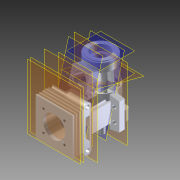
# Autodesk Inventor part: Engine Block
Saved by Autodesk Inventor 2015 (Build 190159000, 159)
## iProperties
Created: 2016-02-24
Part Number: Engine Block
Material: Aluminum 6061-AHC
Document SubType Name: Modeling
Designer: Owner
Density: 2.7 g/cm^3
Appearance: Aluminum - Dark
Author: Owner
Autodesk Inventor part; units mm, degrees
(part 1 of 2)
ref_plane "YZ Plane" through (0, 0, 0) normal (1, 0, 0) x (0, 1, 0)
ref_plane "XZ Plane" through (0, 0, 0) normal (0, 1, 0) x (-1, 0, 0)
sketch "Sketch1" plane through (0, 0, 0) normal (0, 1, 0) x (-1, 0, 0)
  circle A0 centre (0, 0) radius 12.5095
  dimension "d0" = 25.019
  constraints: 1 centre point, 1 coincident
  measures "d0" diameter of A0
extrude "Extrusion1" add sketch "Sketch1" along normal blind 26.162
ref_plane "Work Plane1" through (0, 47.625, 0) normal (0, -1, 0) x (1, 0, 0)
sketch "Sketch2" plane through (0, 47.625, 0) normal (0, -1, 0) x (1, 0, 0)
  circle A0 centre (0, 0) radius 11.049
  dimension "d4" = 22.098
  constraints: 1 centre point, 1 coincident
  measures "d4" diameter of A0
extrude "Extrusion2" add sketch "Sketch2" along normal blind 7.62
sketch "Sketch4" plane through (0, 40.005, 0) normal (0, -1, 0) x (1, 0, 0)
  circle A0 centre (0, 0) radius 7.239
  dimension "d7" = 14.478
  constraints: 1 centre point, 1 coincident
  measures "d7" diameter of A0
sketch "Sketch5" plane through (0, 26.162, 0) normal (0, 1, 0) x (1, 0, 0)
  circle A0 centre (0, 0) radius 8.7122
  dimension "d8" = 17.4244
  constraints: 1 centre point, 1 coincident
  measures "d8" diameter of A0
loft "Loft1" add profiles "Sketch5", "Sketch4"
sketch "Sketch6" plane through (0, 40.005, 0) normal (0, -1, 0) x (1, 0, 0)
  circle A0 centre (0, 0) radius 10.414
  dimension "d13" = 20.828
  constraints: 1 centre point, 1 coincident
  measures "d13" diameter of A0
sketch "Sketch7" plane through (0, 26.162, 0) normal (0, 1, 0) x (1, 0, 0)
  circle A0 centre (0, 0) radius 11.8872
  dimension "d14" = 23.7744
  constraints: 1 centre point, 1 coincident
  measures "d14" diameter of A0
surface_loft "LoftSrf1"
sketch "Sketch8" plane through (0, 0, 0) normal (1, 0, 0) x (0, 1, 0)
  line L0 (47.625, -11.049) -> (40.005, -11.049) construction
  line L1 (40.005, -11.049) -> (40.005, -10.16) construction
  line L2 (40.005, 11.049) -> (40.005, -11.049) construction
  line L3 (40.005, -10.16) -> (26.162, -10.16)
  line L4 (26.162, -12.5095) -> (26.162, 12.5095) projected
  line L5 (40.005, -10.16) -> (40.005, -8.255)
  line L6 (40.005, -8.255) -> (26.162, -8.255)
  line L7 (40.005, -8.255) -> (40.005, -5.08) construction
  line L8 (40.005, -5.08) -> (26.162, -5.08)
  line L9 (26.162, -8.255) -> (26.162, -10.16)
  line L10 (40.005, -5.08) -> (40.005, -3.175)
  line L11 (40.005, -3.175) -> (26.162, -3.175)
  line L12 (26.162, -3.175) -> (26.162, -5.08)
  line L13 (40.005, 0) -> (40.005, 1.905)
  line L14 (40.005, 0) -> (26.162, 0)
  line L15 (26.162, 0) -> (26.162, 1.905)
  line L16 (40.005, 1.905) -> (26.162, 1.905)
  line L17 (40.005, 1.905) -> (40.005, 5.08) construction
  line L18 (40.005, 5.08) -> (26.162, 5.08)
  line L19 (26.162, 5.08) -> (26.162, 6.985)
  line L20 (26.162, 6.985) -> (40.005, 6.985)
  line L21 (40.005, 5.08) -> (40.005, 6.985)
  point P0 (0, 0)
  dimension "d19" = 0.889
  dimension "d20" = 1.905
  dimension "d21" = 3.175
  dimension "d22" = 1.905
  dimension "d23" = 1.905
  dimension "d24" = 3.175
  dimension "d25" = 1.905
  constraints: 38 end point, 6 horizontal, 3 vertical, 1 perpendicular, 1 point on line, 18 other
  measures "d19" distance of L1.start L1.end
  measures "d20" distance of L1.end L5.end
  measures "d21" distance of L5.end L7.end
  measures "d22" distance of L7.end L10.end
  measures "d23" distance of L13.start L13.end
  measures "d24" distance of L13.end L17.end
  measures "d25" distance of L18.end L19.end
extrude "Extrusion3" add sketch "Sketch8" along normal up to surface round surface about axis through (0, 26.162, 0) along (0, 1, 0) radius 11.8872 half angle -6.074668 far side no
mirror "Mirror1" about plane through (0, 0, 0) normal (1, 0, 0) of "Extrusion3"
sketch "Sketch11" plane through (6.1709, 26.162, -10.16) normal (0, 0, -1) x (-1, 0, 0)
  line L0 (12.5196, 13.843) -> (-0.1778, 13.843) projected
  line L1 (6.1709, 13.843) -> (6.1709, 0)
  line L2 (0.964, 0) -> (11.3778, 0) projected
  line L3 (7.4409, 13.843) -> (7.4409, 0)
  line L4 (4.9009, 13.843) -> (4.9009, 0)
  line L5 (4.9009, 13.843) -> (6.1709, 13.843)
  line L6 (6.1709, 13.843) -> (7.4409, 13.843)
  line L7 (6.1709, 0) -> (7.4409, 0)
  line L8 (4.9009, 0) -> (6.1709, 0)
  point P0 (6.1709, -26.162)
  dimension "d30" = 1.27
  dimension "d31" = 1.27
  constraints: 14 end point, 4 collinear, 4 point on line, 2 midpoint, 2 parallel
  measures "d30" distance between parallel lines of L3 L1
  measures "d31" distance between parallel lines of L1 L4
extrude "Extrusion5" add sketch "Sketch11" along normal up to surface from surface at -17.145 round surface about axis through (0, 26.162, 0) along (0, 1, 0) radius 11.8872 half angle -6.074668 far side no
ref_plane "Work Plane2" through (0, 31.75, 0) normal (0, -1, 0) x (1, 0, 0)
ref_plane "Work Plane3" through (0, 31.75, 0) normal (0, -0.258819, -0.9659258) x (1, 0, 0)
ref_plane "Work Plane4" through (0, 31.75, 0) normal (0, 0.9659258, -0.258819) x (1, 0, 0)
ref_plane "Work Plane5" through (0, 0, 20.32) normal (0, 0, 1) x (1, 0, 0)
ref_plane "Work Plane6" through (0, 36.457, 17.5667) normal (0, -0.258819, -0.9659258) x (1, 0, 0)
sketch "Sketch12" plane through (0, 36.457, 17.5667) normal (0, -0.258819, -0.9659258) x (1, 0, 0)
  point P0 (0, 30.6681)
sketch "Sketch13" plane through (0, 36.457, 17.5667) normal (0, -0.258819, -0.9659258) x (1, 0, 0)
  line L0 (-6.985, -6.985) -> (6.985, -6.985)
  line L1 (6.985, -6.985) -> (6.985, 6.985)
  line L2 (6.985, 6.985) -> (-6.985, 6.985)
  line L3 (-6.985, 6.985) -> (-6.985, -6.985)
  line L4 (-6.985, -6.985) -> (6.985, 6.985) construction
  line L5 (6.985, -6.985) -> (-6.985, 6.985) construction
  point P0 (0, 30.6681)
  point P1 (0, 0)
  dimension "d41" = 13.97
  dimension "d42" = 13.97
  constraints: 12 end point, 2 midpoint, 2 parallel, 1 horizontal, 1 perpendicular
  measures "d41" distance of L2.end L1.end
  measures "d42" distance of L1.end L0.end
extrude "Extrusion6" add sketch "Sketch13" along normal up to next
sketch "Sketch14" plane through (0, 0, 0) normal (0, -1, 0) x (1, 0, 0)
  line L0 (9.0932, -9.0932) -> (-9.0932, -9.0932)
  line L1 (-9.0932, -9.0932) -> (-9.0932, 9.0932)
  line L2 (-9.0932, 9.0932) -> (9.0932, 9.0932)
  line L3 (9.0932, 9.0932) -> (9.0932, -9.0932)
  line L4 (9.0932, -9.0932) -> (-9.0932, 9.0932) construction
  line L5 (-9.0932, -9.0932) -> (9.0932, 9.0932) construction
  circle A0 centre (9.0932, -9.0932) radius 3.175
  circle A1 centre (-9.0932, -9.0932) radius 3.175
  circle A2 centre (-9.0932, 9.0932) radius 3.175
  circle A3 centre (9.0932, 9.0932) radius 3.175
  point P0 (0, 0)
  dimension "d45" = 18.1864
  dimension "d46" = 18.1864
  dimension "d47" = 6.35
  dimension "d48" = 6.35
  dimension "d49" = 6.35
  dimension "d50" = 6.35
  constraints: 12 end point, 4 centre point, 4 coincident, 2 midpoint, 2 parallel, 1 horizontal, 1 perpendicular
  measures "d45" distance of L1.end L2.end
  measures "d46" distance of L0.end L1.end
  measures "d47" diameter of A0
  measures "d48" diameter of A1
  measures "d49" diameter of A2
  measures "d50" diameter of A3
extrude "Extrusion7" add sketch "Sketch14" against normal blind 8.128 contours A1 L1 L0 | L0 L1 A1 | A0 L3 L0 | L0 L3 A0 | A2 L2 L1 | L1 L2 A2 | A3 L2 L3 | L3 L2 A3
sketch "Sketch15" plane through (0, 0, 0) normal (0, -1, 0) x (1, 0, 0)
  arc A0 (6.3881, -10.7555) -> (10.7555, -6.3881) centre (9.0932, -9.0932) ccw projected
  arc A1 (-10.7555, -6.3881) -> (-6.3881, -10.7555) centre (-9.0932, -9.0932) ccw projected
  arc A2 (-6.3881, 10.7555) -> (-10.7555, 6.3881) centre (-9.0932, 9.0932) ccw projected
  arc A3 (10.7555, 6.3881) -> (6.3881, 10.7555) centre (9.0932, 9.0932) ccw projected
  point P0 (0, 0)
hole "Hole1" at (9.0932, 0, -9.0932) at (-9.0932, 0, -9.0932) at (-9.0932, 0, 9.0932) at (9.0932, 0, 9.0932) direction (0, 1, 0) diameter 1.9304 depth 5.715 tip angle 118
fillet "Fillet1" radius 5.08 4 edges at (6.3881, 4.064, 10.7555) (-6.3881, 4.064, 10.7555) (-6.3881, 4.064, -10.7555) (6.3881, 4.064, -10.7555)
sketch "Sketch16" plane through (0, 0, 0) normal (0, 0, 1) x (1, 0, 0)
  line L0 (4.0733, 0) -> (4.0733, 8.128) projected
  line L1 (-4.0733, 0) -> (4.0733, 0) projected
  line L2 (-4.0733, 8.128) -> (-4.0733, 0) projected
  line L3 (-4.0733, 8.128) -> (-10.7555, 8.128) projected
  line L4 (-10.7555, 8.128) -> (-10.7555, 0) projected
  line L5 (-10.7555, 0) -> (-10.7555, 0) projected
  line L6 (-10.7555, 0) -> (-10.7555, 8.128) projected
  line L7 (-10.7555, 8.128) -> (-4.0733, 8.128) projected
  line L8 (-4.0733, 0) -> (-4.0733, 8.128) projected
  line L9 (4.0733, 0) -> (-4.0733, 0) projected
  line L10 (4.0733, 8.128) -> (4.0733, 0) projected
  line L11 (4.0733, 8.128) -> (10.7555, 8.128) projected
  line L12 (10.7555, 8.128) -> (10.7555, 0) projected
  line L13 (10.7555, 0) -> (10.7555, 0) projected
  line L14 (10.7555, 0) -> (10.7555, 8.128) projected
  line L15 (10.7555, 8.128) -> (4.0733, 8.128) projected
  line L16 (12.5095, 26.162) -> (-12.5095, 26.162) projected
  line L17 (-12.5095, 0) -> (-12.5095, 26.162) projected
  line L18 (-7.7987, 0) -> (-12.2682, 0) projected
  line L19 (-7.7987, 0) -> (-4.0733, 0) projected
  line L20 (12.5095, 0) -> (12.5095, 26.162) projected
  line L21 (-12.5095, 0) -> (-6.9215, 0)
  line L22 (-6.9215, 0) -> (-6.9215, 26.162)
  line L23 (-7.0779, 26.162) -> (-2.7852, 26.162) projected
  line L24 (-6.9215, 0) -> (-19.4918, 2.2844)
  line L25 (-6.9215, 0) -> (5.8547, 0) construction
  line L26 (-19.4918, 2.2844) -> (-19.4918, 23.8744)
  line L27 (-19.4918, 23.8744) -> (-6.9215, 26.162)
  point P0 (0, 0)
  dimension "d61" = 5.588
  dimension "d62" = 12.7762
  dimension "d63" = 169.7
  dimension "d64" = 21.59
  constraints: 12 end point, 2 point on line, 1 equal length, 1 horizontal, 1 perpendicular, 1 vertical
  measures "d61" distance of L17.start L21.end
  measures "d62" distance of L21.end L24.end
  measures "d63" angle of L25 L24
  measures "d64" distance of L24.end L26.end
extrude "Extrusion8" add sketch "Sketch16" along normal blind 4.445 contours L22 L24 L4 L3 | L3 L4 L24 L17 L27 L22 | L17 L24 L26 L27
sketch "Sketch17" plane through (0, 0, 0) normal (0, 0, 1) x (1, 0, 0)
  line L0 (-19.4918, 2.2844) -> (-15.6818, 2.2844) construction
  line L1 (-19.4918, 2.2844) -> (-12.5095, 1.0155) projected
  line L2 (-19.4918, 23.8744) -> (-19.4918, 2.2844) projected
  line L3 (-19.4918, 2.2844) -> (-11.6931, 0.8672) projected
  line L4 (-15.5925, 1.5758) -> (-15.5925, 7.4686) construction
  line L5 (-15.5925, 7.4686) -> (-15.5925, 18.2636)
  line L6 (-15.5925, 12.8661) -> (-19.4918, 12.8661)
  circle A0 centre (-15.5925, 7.4686) radius 1.5875
  circle A1 centre (-15.5925, 18.2636) radius 1.5875
  point P0 (0, 0)
  dimension "d67" = 3.81
  dimension "d68" = 5.8928
  dimension "d69" = 10.795
  dimension "d70" = 3.175
  dimension "d71" = 3.175
  constraints: 8 end point, 2 centre point, 2 coincident, 2 midpoint, 2 vertical, 1 horizontal, 1 perpendicular, 1 point on line
  measures "d67" distance of L0.start L0.end
  measures "d68" distance of L4.start L4.end
  measures "d69" distance of L4.end L5.end
  measures "d70" diameter of A0
  measures "d71" diameter of A1
hole "Hole2" at (-15.5925, 7.4686, 0) at (-15.5925, 18.2636, 0) direction (0, 0, 1) diameter 3.175 end through all
mirror "Mirror2" about plane through (0, 0, 0) normal (1, 0, 0) of "Extrusion8", "Hole2"
ref_plane "Work Plane7" through (0, 0, 37.592) normal (0, 0, 1) x (1, 0, 0)
sketch "Sketch18" plane through (0, 0, 37.592) normal (0, 0, 1) x (1, 0, 0)
  line L0 (11.6931, 25.2936) -> (12.5095, 25.1451) projected
  line L1 (12.5095, 25.1451) -> (12.5095, 1.0155) projected
  line L2 (12.5095, 1.0155) -> (11.6931, 0.8672) projected
  line L3 (11.6931, 0.8672) -> (11.6931, 25.2936) projected
  line L4 (-12.5095, 25.1451) -> (-11.6931, 25.2936) projected
  line L5 (-11.6931, 25.2936) -> (-11.6931, 0.8672) projected
  line L6 (-11.6931, 0.8672) -> (-12.5095, 1.0155) projected
  line L7 (-12.5095, 1.0155) -> (-12.5095, 25.1451) projected
  line L8 (4.0733, 0) -> (4.0733, 8.128) projected
  line L9 (-4.0733, 0) -> (4.0733, 0) projected
  line L10 (-4.0733, 8.128) -> (-4.0733, 0) projected
  line L11 (-4.0733, 8.128) -> (-10.7555, 8.128) projected
  line L12 (-10.7555, 8.128) -> (-10.7555, 0) projected
  line L13 (-10.7555, 0) -> (-10.7555, 0) projected
  line L14 (-10.7555, 0) -> (-10.7555, 8.128) projected
  line L15 (-10.7555, 8.128) -> (-4.0733, 8.128) projected
  line L16 (-4.0733, 0) -> (-4.0733, 8.128) projected
  line L17 (4.0733, 0) -> (-4.0733, 0) projected
  line L18 (4.0733, 8.128) -> (4.0733, 0) projected
  line L19 (4.0733, 8.128) -> (10.7555, 8.128) projected
  line L20 (10.7555, 8.128) -> (10.7555, 0) projected
  line L21 (10.7555, 0) -> (10.7555, 0) projected
  line L22 (10.7555, 0) -> (10.7555, 8.128) projected
  line L23 (10.7555, 8.128) -> (4.0733, 8.128) projected
  line L24 (12.5095, 26.162) -> (-12.5095, 26.162) projected
  line L25 (10.668, 0.6343) -> (-10.668, 0.6343)
  line L26 (-10.668, 0.6343) -> (-10.668, 25.5263)
  line L27 (-10.668, 25.5263) -> (10.668, 25.5263)
  line L28 (10.668, 25.5263) -> (10.668, 0.6343)
  line L29 (10.668, 0.6343) -> (-10.668, 25.5263) construction
  line L30 (-10.668, 0.6343) -> (10.668, 25.5263) construction
  point P0 (0, 0)
  point P1 (0, 13.0803)
  dimension "d80" = 21.336
  dimension "d81" = 24.892
  constraints: 12 end point, 2 midpoint, 2 parallel, 1 horizontal, 1 perpendicular
  measures "d80" distance of L26.end L27.end
  measures "d81" distance of L25.end L26.end
extrude "Extrusion9" add sketch "Sketch18" against normal up to next contours L25 L10 L11 L26 L27 L28 L19 L8 | L8 L19 L28 L25 | L25 L26 L11 L10
sketch "Sketch20" plane through (0, 0, 0) normal (1, 0, 0) x (0, 1, 0)
  line L0 (26.162, -12.5095) -> (26.162, 12.5095) projected
  line L1 (8.128, -6.3881) -> (8.128, -11.8277) projected
  line L2 (0, -11.8277) -> (8.128, -11.8277) projected
  line L3 (0, -11.8277) -> (0, -11.8277) projected
  line L4 (8.128, -11.8277) -> (0, -11.8277) projected
  line L5 (8.128, -11.8277) -> (8.128, -6.3881) projected
  line L6 (8.128, -6.3881) -> (0, -6.3881) projected
  line L7 (0, 6.3881) -> (0, -6.3881) projected
  line L8 (0, 6.3881) -> (8.128, 6.3881) projected
  line L9 (8.128, 6.3881) -> (8.128, 6.5331) projected
  line L10 (8.128, 6.5331) -> (25.5263, 6.5331) projected
  line L11 (25.5263, 6.5331) -> (25.5263, 6.5331) projected
  line L12 (25.5263, 6.5331) -> (8.128, 6.5331) projected
  line L13 (8.128, 6.5331) -> (8.128, 6.3881) projected
  line L14 (8.128, 6.3881) -> (0, 6.3881) projected
  line L15 (0, -6.3881) -> (0, 6.3881) projected
  line L16 (0, -6.3881) -> (8.128, -6.3881) projected
  ellipse E0 centre (27.4216, 0) end of major axis (27.4216, -12.5095) minor radius 2.2765 (25.2936, 4.445) -> (25.1451, 0) ccw projected
  line L17 (25.2936, 4.445) -> (0.8672, 4.445) projected
  ellipse E1 centre (-1.2578, 0) end of major axis (-1.2578, 12.5095) minor radius 2.2734 (1.0155, 0) -> (0.8672, 4.445) ccw projected
  line L18 (1.0155, 0) -> (25.1451, 0) projected
  ellipse E2 centre (27.4216, 0) end of major axis (27.4216, -12.5095) minor radius 2.2765 (25.2936, 4.445) -> (25.1451, 0) ccw projected
  line L19 (25.1451, 0) -> (1.0155, 0) projected
  ellipse E3 centre (-1.2578, 0) end of major axis (-1.2578, 12.5095) minor radius 2.2734 (1.0155, 0) -> (0.8672, 4.445) ccw projected
  line L20 (0.8672, 4.445) -> (25.2936, 4.445) projected
  line L21 (8.128, 6.5331) -> (25.5263, 6.5331) projected
  line L22 (8.128, 11.8501) -> (8.128, 6.5331) projected
  line L23 (0.6343, 11.8501) -> (8.128, 11.8501) projected
  line L24 (0.6343, 37.592) -> (0.6343, 11.8501) projected
  line L25 (0.6343, 37.592) -> (25.5263, 37.592) projected
  line L26 (25.5263, 37.592) -> (25.5263, 6.5331) projected
  line L27 (26.162, 5.08) -> (26.162, 1.905) projected
  line L28 (26.162, 4.445) -> (13.081, 4.445)
  line L29 (23.8744, 4.445) -> (2.2844, 4.445) projected
  line L30 (13.081, 4.445) -> (13.081, 12.065) construction
  line L31 (5.461, 4.445) -> (20.701, 4.445)
  line L32 (20.701, 4.445) -> (20.701, 19.685)
  line L33 (20.701, 19.685) -> (5.461, 19.685)
  line L34 (5.461, 19.685) -> (5.461, 4.445)
  line L35 (5.461, 4.445) -> (20.701, 19.685) construction
  line L36 (20.701, 4.445) -> (5.461, 19.685) construction
  point P0 (0, 0)
  dimension "d88" = 13.081
  dimension "d89" = 7.62
  dimension "d90" = 15.24
  dimension "d91" = 15.24
  constraints: 16 end point, 2 midpoint, 2 parallel, 2 perpendicular, 2 point on line, 1 horizontal, 4 other
  measures "d88" distance of L28.start L28.end
  measures "d89" distance of L28.end L30.end
  measures "d90" distance of L33.end L32.end
  measures "d91" distance of L32.end L31.end
extrude "Extrusion10" add sketch "Sketch20" along normal mid plane 25.4 contours L34 L23 L22 L9 L8 | L8 L9 L10 L32 L17 L34 | L34 L33 L32 L10 L22 L23
chamfer "Chamfer1" distance 3.175 angle 45 4 edges at (-10.668, 0.6343, 24.7211) (10.668, 0.6343, 24.7211) (-10.668, 25.5263, 22.0625) (10.668, 25.5263, 22.0625)
sketch "Sketch21" plane through (0, 0, 37.592) normal (0, 0, 1) x (1, 0, 0)
  line L0 (0, 0) -> (0, 13.081) construction
  line L1 (-14.986, 28.321) -> (14.986, 28.321)
  line L2 (14.986, 28.321) -> (14.986, -2.159)
  line L3 (14.986, -2.159) -> (-14.986, -2.159)
  line L4 (-14.986, -2.159) -> (-14.986, 28.321)
  line L5 (-14.986, 28.321) -> (14.986, -2.159) construction
  line L6 (14.986, 28.321) -> (-14.986, -2.159) construction
  dimension "d97" = 13.081
  dimension "d98" = 29.972
  dimension "d99" = 30.48
  constraints: 14 end point, 2 midpoint, 2 parallel, 1 horizontal, 1 perpendicular, 1 vertical
  measures "d97" distance of L0.start L0.end
  measures "d98" distance of L2.end L3.end
  measures "d99" distance of L1.end L2.end
extrude "Extrusion11" add sketch "Sketch21" against normal blind 15.24
ref_plane "Work Plane8" through (0, 0, 35.052) normal (0, 0, 1) x (1, 0, 0)
sketch "Sketch22" plane through (0, 0, 35.052) normal (0, 0, 1) x (1, 0, 0)
  line L0 (0, 0) -> (0, 13.081)
  line L1 (-8.636, 21.971) -> (8.636, 21.971)
  line L2 (8.636, 21.971) -> (8.636, 4.191)
  line L3 (8.636, 4.191) -> (-8.636, 4.191)
  line L4 (-8.636, 4.191) -> (-8.636, 21.971)
  line L5 (-8.636, 21.971) -> (8.636, 4.191) construction
  line L6 (8.636, 21.971) -> (-8.636, 4.191) construction
  line L7 (-10.668, 20.701) -> (-10.668, 5.461)
  line L8 (-10.668, 20.701) -> (-10.668, 5.461) projected
  line L9 (10.668, 5.461) -> (10.668, 20.701) projected
  line L10 (-7.7987, 0) -> (-4.0733, 0) projected
  line L11 (-7.7987, 0) -> (-12.2682, 0) projected
  line L12 (-12.2682, 0) -> (-12.2682, 8.128) projected
  line L13 (12.2682, 0) -> (7.7987, 0) projected
  line L14 (4.0733, 0) -> (7.7987, 0) projected
  line L15 (7.7987, 0.94) -> (10.668, 3.8093) projected
  line L16 (-7.7987, 0.94) -> (-10.668, 3.8093) projected
  line L17 (10.668, 20.701) -> (10.668, 22.3513)
  line L18 (10.668, 22.3513) -> (7.493, 25.5263)
  line L19 (7.493, 25.5263) -> (10.668, 22.3513) projected
  line L20 (7.493, 25.5263) -> (-7.493, 25.5263)
  line L21 (-7.493, 25.5263) -> (7.493, 25.5263) projected
  line L22 (-7.493, 25.5263) -> (-10.668, 22.3513)
  line L23 (-10.668, 22.3513) -> (-7.493, 25.5263) projected
  line L24 (-10.668, 22.3513) -> (-10.668, 3.8093)
  line L25 (-10.668, 3.8093) -> (-10.668, 22.3513) projected
  line L26 (-10.668, 3.8093) -> (-7.493, 0.6343)
  line L27 (-7.493, 0.6343) -> (-10.668, 3.8093) projected
  line L28 (-7.493, 0.6343) -> (7.493, 0.6343)
  line L29 (7.493, 0.6343) -> (10.668, 3.8093)
  line L30 (10.668, 3.8093) -> (10.668, 22.3513)
  line L31 (14.986, 28.321) -> (-14.986, 28.321)
  line L32 (-14.986, 28.321) -> (-14.986, -2.159)
  line L33 (-14.986, -2.159) -> (-14.986, 28.321) projected
  line L34 (-14.986, -2.159) -> (14.986, -2.159)
  line L35 (14.986, -2.159) -> (14.986, 28.321)
  line L36 (14.986, 28.321) -> (14.986, -2.159) projected
  dimension "d103" = 13.081
  dimension "d104" = 17.272
  dimension "d105" = 17.78
  constraints: 42 end point, 9 collinear, 3 parallel, 3 perpendicular, 2 horizontal, 2 midpoint, 2 vertical
  measures "d103" distance of L0.start L0.end
  measures "d104" distance of L2.end L3.end
  measures "d105" distance of L1.end L2.end
extrude "Extrusion12" cut sketch "Sketch22" along normal blind 1.27 contours L35 L34 L32 L31
pattern_linear "Rectangular Pattern1" count 6 spacing 2.54 along (0, 0, -1) of "Extrusion12"
sketch "Sketch24" plane through (14.986, -2.159, 28.702) normal (1, 0, 0) x (0, 0, -1)
  line L0 (0, 0) -> (0, 30.48)
  line L1 (0, 30.48) -> (6.35, 30.48) construction
  line L2 (3.81, 30.48) -> (5.08, 30.48) projected
  line L3 (6.35, 30.48) -> (6.35, 0)
  arc A0 (6.35, 30.48) -> (0, 30.48) centre (3.175, 30.48) ccw
  arc A1 (0, 0) -> (6.35, 0) centre (3.175, 0) ccw
  line L4 (0, 30.48) -> (-1.27, 30.48)
  line L5 (-1.27, 30.48) -> (-1.27, 0)
  line L6 (-1.27, 0) -> (0, 0)
  point P0 (28.702, 2.159)
  dimension "d111" = 6.35
  constraints: 12 end point, 4 point on circle, 4 tangent, 3 perpendicular, 2 centre point, 1 collinear, 1 horizontal, 1 vertical
  measures "d111" distance of L0.end L1.end
extrude "Extrusion13" add sketch "Sketch24" against normal up to surface (14.986 mm away)
sketch "Sketch26" plane through (0, 0, 0) normal (0, -1, 0) x (1, 0, 0)
  arc A0 (10.7555, -6.3881) -> (10.7555, 6.3881) centre (0, 0) ccw projected
hole "Hole3" at (0, 0, 0) direction (0, 1, 0) diameter 20.955 depth 19.685
sketch "Sketch27" plane through (0, 0, 37.592) normal (0, 0, 1) x (1, 0, 0)
  line L0 (14.986, 28.321) -> (14.986, -2.159) projected
  line L1 (-14.986, -2.159) -> (-14.986, 28.321) projected
  line L2 (14.986, -2.159) -> (-14.986, -2.159) projected
  line L3 (-14.986, 28.321) -> (14.986, 28.321) projected
  line L4 (8.4836, 4.5974) -> (-8.4836, 4.5974)
  line L5 (-8.4836, 4.5974) -> (-8.4836, 21.5646)
  line L6 (-8.4836, 21.5646) -> (8.4836, 21.5646)
  line L7 (8.4836, 21.5646) -> (8.4836, 4.5974)
  line L8 (8.4836, 4.5974) -> (-8.4836, 21.5646) construction
  line L9 (-8.4836, 4.5974) -> (8.4836, 21.5646) construction
  point P0 (0, 0)
  point P1 (0, 13.081)
  dimension "d121" = 16.9672
  dimension "d122" = 16.9672
  constraints: 12 end point, 2 midpoint, 2 parallel, 1 horizontal, 1 perpendicular
  measures "d121" distance of L5.end L6.end
  measures "d122" distance of L4.end L5.end
hole "Hole4" at (8.4836, 21.5646, 37.592) at (8.4836, 4.5974, 37.592) at (-8.4836, 4.5974, 37.592) at (-8.4836, 21.5646, 37.592) direction (0, 0, -1) diameter 1.9304 depth 7.62 tip angle 118
sketch "Sketch28" plane through (0, 0, 37.592) normal (0, 0, 1) x (1, 0, 0)
  circle A0 centre (8.4836, 21.5646) radius 0.9652 projected
  circle A1 centre (-8.4836, 4.5974) radius 0.9652 projected
  line L0 (8.4836, 21.5646) -> (-8.4836, 4.5974) construction
  circle A2 centre (-8.4836, 21.5646) radius 0.9652 projected
  line L1 (-8.4836, 21.5646) -> (8.4836, 4.5974)
  line L2 (-8.4836, 21.5646) -> (15.5116, 21.5646) construction
  circle A3 centre (-8.4836, 4.5974) radius 0.9652 projected
  circle A4 centre (8.4836, 21.5646) radius 0.9652 projected
  circle A5 centre (8.4836, 4.5974) radius 0.9652 projected
  circle A6 centre (-8.4836, 21.5646) radius 0.9652 projected
  line L3 (-14.986, 28.321) -> (14.986, 28.321) projected
  line L4 (-14.986, -2.159) -> (-14.986, 28.321) projected
  line L5 (14.986, -2.159) -> (-14.986, -2.159) projected
  line L6 (14.986, 28.321) -> (14.986, -2.159) projected
  circle A7 centre (0, 13.081) radius 9.017
  point P0 (0, 0)
  dimension "d130" = 45
  dimension "d131" = 18.034
  constraints: 6 end point, 1 centre point, 1 equal length, 1 horizontal, 1 midpoint
  measures "d130" angle of L1 L2
  measures "d131" diameter of A7
hole "Hole5" at (0, 13.081, 37.592) direction (0, 0, -1) diameter 18.034 depth 27.559 tip angle 118
sketch "Sketch29" plane through (0, 47.625, 0) normal (0, 1, 0) x (1, 0, 0)
  circle A0 centre (0, 0) radius 9.9695
  circle A1 centre (0, 0) radius 11.049 projected
  dimension "d139" = 19.939
  constraints: 1 centre point, 1 coincident
  measures "d139" diameter of A0
extrude "Extrusion14" cut sketch "Sketch29" against normal blind 0.635
sketch "Sketch30" plane through (0, 47.625, 0) normal (0, 1, 0) x (1, 0, 0)
  circle A0 centre (0, 0) radius 9.9695 projected
hole "Hole6" at (0, 47.625, 0) direction (0, -1, 0) diameter 13.97 depth 5.08
sketch "Sketch31" plane through (0, 19.685, 0) normal (0, -1, 0) x (1, 0, 0)
  arc A0 (-4.5551, 9.4355) -> (4.5551, 9.4355) centre (0, 0) ccw projected
  constraints: 1 horizontal alignment
hole "Hole7" at (0, 19.685, 0) direction (0, 1, 0) diameter 13.97 depth 5.08
sketch "Sketch32" plane through (0, 42.545, 0) normal (0, 1, 0) x (1, 0, 0)
  circle A0 centre (0, 0) radius 6.985 projected
hole "Hole8" at (0, 42.545, 0) direction (0, -1, 0) diameter 9.017 end through all
sketch "Sketch33" plane through (-6.985, 26.3902, 6.985) normal (-1, 0, 0) x (0, 0, 1)
  line L0 (12.3896, 3.3198) -> (7.9446, 3.3198)
  circle A0 centre (7.9446, 3.3198) radius 3.4925
  point P0 (-6.985, -26.3902)
  dimension "d163" = 4.445
  dimension "d164" = 6.985
  constraints: 2 end point, 1 centre point, 1 coincident, 1 horizontal
  measures "d163" distance of L0.start L0.end
  measures "d164" diameter of A0
extrude "Extrusion15" add sketch "Sketch33" against normal up to surface (13.97 mm away)
sketch "Sketch34" plane through (-6.985, 26.3902, 6.985) normal (-1, 0, 0) x (0, 0, 1)
  line L0 (12.3896, 3.3198) -> (11.4275, 3.062) projected
  line L1 (12.3896, 3.3198) -> (8.7739, 16.8138) projected
  line L2 (8.7739, 16.8138) -> (1.576, 14.8851) projected
  line L3 (1.576, 13.6148) -> (1.576, 14.8851) projected
  line L4 (0, 13.6148) -> (1.576, 13.6148) projected
  line L5 (0, 0) -> (0, 13.6148) projected
  line L6 (5.0571, 1.355) -> (0, 0) projected
  arc A0 (5.0571, 1.355) -> (11.4275, 3.062) centre (7.9446, 3.3198) ccw projected
  circle A1 centre (7.9446, 3.3198) radius 3.4925
  point P0 (-6.985, -26.3902)
  constraints: 1 centre point, 1 coincident
extrude "Extrusion16" add sketch "Sketch34" along normal blind 0.635 contours A0 A1
sketch "Sketch35" plane through (6.985, 26.3902, 6.985) normal (1, 0, 0) x (0, 0, -1)
  line L0 (-5.0571, 1.355) -> (0, 0) projected
  line L1 (0, 13.6148) -> (0, 0) projected
  line L2 (-1.576, 13.6148) -> (0, 13.6148) projected
  line L3 (-1.576, 14.8851) -> (-1.576, 13.6148) projected
  line L4 (-8.7739, 16.8138) -> (-1.576, 14.8851) projected
  line L5 (-8.7739, 16.8138) -> (-12.3896, 3.3198) projected
  line L6 (-12.3896, 3.3198) -> (-11.4275, 3.062) projected
  arc A0 (-11.4275, 3.062) -> (-5.0571, 1.355) centre (-7.9446, 3.3198) ccw projected
  circle A1 centre (-7.9446, 3.3198) radius 3.4925
  point P0 (6.985, -26.3902)
  constraints: 1 centre point, 1 coincident
extrude "Extrusion17" add sketch "Sketch35" along normal blind 0.635 contours A0 A1
sketch "Sketch36" plane through (7.62, 29.71, 14.9296) normal (1, 0, 0) x (0, 0, -1)
  circle A0 centre (0, 0) radius 3.4925 projected
  point P0 (14.9296, -29.71)
hole "Hole9" at (7.62, 29.71, 14.9296) direction (-1, 0, 0) diameter 3.937 end through all
sketch "Sketch37" plane through (14.986, -2.159, 29.972) normal (1, 0, 0) x (0, 0, -1)
  line L0 (0, 30.48) -> (1.27, 30.48) projected
  line L1 (0, 30.48) -> (0, 0) projected
  line L2 (0, 0) -> (1.27, 0) projected
  arc A0 (1.27, 0) -> (7.62, 0) centre (4.445, 0) ccw projected
  line L3 (7.62, 0) -> (7.62, 30.48) projected
  arc A1 (7.62, 30.48) -> (1.27, 30.48) centre (4.445, 30.48) ccw projected
  point P0 (29.972, 2.159)
hole "Hole10" at (14.986, 28.321, 25.527) at (14.986, -2.159, 25.527) direction (-1, 0, 0) diameter 3.2766 end through all clearance for "Flat Head Machine Screw (82)" size "#4" standard "Ansi Unified Screw Threads"
ref_plane "Work Plane11" through (0, 0, 23.9014) normal (0, 0, 1) x (1, 0, 0)
sketch "Sketch39" plane through (0, 31.75, 0) normal (0, -1, 0) x (1, 0, 0)
  point P0 (0, 0)
sketch "Sketch40" plane through (0, 36.457, 17.5667) normal (0, 0.258819, 0.9659258) x (1, 0, 0)
  circle A0 centre (0, 0) radius 6.223
  point P0 (0, -30.6681)
  dimension "d196" = 12.446
  constraints: 1 centre point
  measures "d196" diameter of A0
hole "Hole12" at (0, 36.457, 17.5667) direction (0, -0.258819, -0.9659258) diameter 12.446 depth 0.762
sketch "Sketch41" plane through (0, 36.2598, 16.8307) normal (0, 0.258819, 0.9659258) x (1, 0, 0)
  circle A0 centre (0, 0) radius 6.223 projected
  point P0 (0, -30.6681)
hole "Hole13" at (0, 36.2598, 16.8307) direction (0, -0.258819, -0.9659258) diameter 9.9568 depth 9.525
sketch "Sketch42" plane through (0, 33.7945, 7.6302) normal (0, 0.258819, 0.9659258) x (1, 0, 0)
  circle A0 centre (0, 0) radius 4.9784
  point P0 (0, -30.6681)
  dimension "d211" = 9.9568
  constraints: 1 centre point
  measures "d211" diameter of A0
hole "Hole14" at (0, 33.7945, 7.6302) direction (0, -0.258819, -0.9659258) diameter 8.89 end up to surface
sketch "Sketch43" plane through (0, 0, 23.9014) normal (0, 0, 1) x (1, 0, 0)
  arc A0 (3.0194, 4.5846) -> (-3.0194, 4.5846) centre (0, 13.081) ccw projected
  line L0 (0, 13.081) -> (9.017, 13.081) construction
  line L1 (9.017, 13.081) -> (14.986, 21.9304)
  line L2 (0, 13.081) -> (11.8449, 13.081) construction
  circle A1 centre (0, 13.081) radius 9.017 projected
  line L3 (0, 4.064) -> (14.986, 4.064)
  line L4 (14.986, -2.159) -> (14.986, 28.321) projected
  circle A2 centre (0, 13.081) radius 9.017
  line L5 (14.986, 21.9304) -> (14.986, 4.064)
  point P0 (0, 0)
  dimension "d219" = 56
  constraints: 10 end point, 3 horizontal, 2 point on circle, 1 centre point, 1 coincident, 1 collinear, 1 point on line, 1 tangent
  measures "d219" angle of L2 L1
extrude "Extrusion18" cut sketch "Sketch43" along normal blind 3.175 contours A0 L1 L4 L3 A1
sketch "Sketch44" plane through (0, 0, 37.592) normal (0, 0, 1) x (1, 0, 0)
  circle A0 centre (0, 13.081) radius 9.017 projected
  line L0 (0, 13.081) -> (7.62, 13.081)
  line L1 (7.62, 13.081) -> (7.62, 6.731)
  circle A1 centre (7.62, 6.731) radius 0.508
  point P0 (0, 0)
  dimension "d222" = 7.62
  dimension "d223" = 6.35
  dimension "d224" = 1.016
  constraints: 4 end point, 1 centre point, 1 coincident, 1 horizontal, 1 vertical
  measures "d222" distance of L0.start L0.end
  measures "d223" distance of L0.end L1.end
  measures "d224" diameter of A1
extrude "Extrusion19" add sketch "Sketch44" along normal blind 0.889 contours A1
sketch "Sketch46" plane through (-12.7, 0, 0) normal (-1, 0, 0) x (0, 0, 1)
  line L0 (18.0769, 21.686) -> (18.0769, 5.0346) construction
  line L1 (18.0769, 5.0346) -> (2.9704, 5.0346) construction
  line L2 (2.9704, 5.0346) -> (2.9704, 21.686) construction
  line L3 (2.9704, 21.686) -> (18.0769, 21.686) construction
  spline S0 degree 2 poles (17.315, 16.7118) (17.1237, 16.7118) (16.8157, 16.8669) (16.7297, 16.9971) knots 0 0 0 1 2 2 2
  spline S1 degree 2 poles (16.7297, 16.9971) (16.6629, 17.1035) (16.6176, 17.322) (16.6176, 17.4919) knots 0 0 0 1 2 2 2
  line L4 (16.6176, 17.4919) -> (16.6176, 17.8134)
  line L5 (16.6176, 17.8134) -> (18.0146, 17.8134)
  line L6 (18.0146, 17.8134) -> (18.0146, 17.4952)
  spline S2 degree 2 poles (18.0146, 17.4952) (18.0146, 17.2983) (17.9557, 17.0741) (17.9037, 16.9949) knots 0 0 0 1 2 2 2
  spline S3 degree 2 poles (17.9037, 16.9949) (17.8142, 16.8601) (17.5188, 16.7118) (17.315, 16.7118) knots 0 0 0 1 2 2 2
  spline S4 degree 2 poles (17.3173, 16.9054) (17.478, 16.9054) (17.7056, 17.0118) (17.7701, 17.1171) knots 0 0 0 1 2 2 2
  spline S5 degree 2 poles (17.7701, 17.1171) (17.8142, 17.1918) (17.8539, 17.3605) (17.8539, 17.4862) knots 0 0 0 1 2 2 2
  line L7 (17.8539, 17.4862) -> (17.8539, 17.6277)
  line L8 (17.8539, 17.6277) -> (16.7784, 17.6277)
  line L9 (16.7784, 17.6277) -> (16.7784, 17.4862)
  spline S6 degree 2 poles (16.7784, 17.4862) (16.7784, 17.3628) (16.818, 17.176) (16.8712, 17.1001) knots 0 0 0 1 2 2 2
  spline S7 degree 2 poles (16.8712, 17.1001) (16.9369, 17.0028) (17.1542, 16.9054) (17.3173, 16.9054) knots 0 0 0 1 2 2 2
  spline S8 degree 2 poles (16.7286, 15.9398) (16.7127, 15.9613) (16.6561, 16.0337) (16.6391, 16.0677) knots 0 0 0 1 2 2 2
  spline S9 degree 2 poles (16.6391, 16.0677) (16.6142, 16.1141) (16.5882, 16.2013) (16.5882, 16.2805) knots 0 0 0 1 2 2 2
  spline S10 degree 2 poles (16.5882, 16.2805) (16.5882, 16.345) (16.6369, 16.4616) (16.681, 16.5058) knots 0 0 0 1 2 2 2
  spline S11 degree 2 poles (16.681, 16.5058) (16.724, 16.5477) (16.8508, 16.5986) (16.921, 16.5986) knots 0 0 0 1 2 2 2
  spline S12 degree 2 poles (16.921, 16.5986) (17.0297, 16.5986) (17.1837, 16.5069) (17.2278, 16.4073) knots 0 0 0 1 2 2 2
  spline S13 degree 2 poles (17.2278, 16.4073) (17.2686, 16.319) (17.2991, 16.079) (17.3071, 15.9398) knots 0 0 0 1 2 2 2
  line L10 (17.3071, 15.9398) -> (17.341, 15.9398)
  spline S14 degree 2 poles (17.341, 15.9398) (17.4022, 15.9398) (17.478, 15.9771) (17.4995, 16.0111) knots 0 0 0 1 2 2 2
  spline S15 degree 2 poles (17.4995, 16.0111) (17.521, 16.045) (17.5346, 16.1424) (17.5346, 16.1945) knots 0 0 0 1 2 2 2
  spline S16 degree 2 poles (17.5346, 16.1945) (17.5346, 16.2556) (17.4984, 16.4209) (17.4633, 16.5035) knots 0 0 0 1 2 2 2
  line L11 (17.4633, 16.5035) -> (17.4633, 16.5137)
  line L12 (17.4633, 16.5137) -> (17.6433, 16.5137)
  spline S17 degree 2 poles (17.6433, 16.5137) (17.6569, 16.465) (17.6908, 16.2828) (17.6908, 16.1933) knots 0 0 0 1 2 2 2
  spline S18 degree 2 poles (17.6908, 16.1933) (17.6908, 16.0847) (17.6569, 15.9364) (17.6127, 15.8775) knots 0 0 0 1 2 2 2
  spline S19 degree 2 poles (17.6127, 15.8775) (17.5697, 15.8198) (17.4327, 15.7631) (17.3342, 15.7631) knots 0 0 0 1 2 2 2
  line L13 (17.3342, 15.7631) -> (16.6176, 15.7631)
  line L14 (16.6176, 15.7631) -> (16.6176, 15.9398)
  line L15 (16.6176, 15.9398) -> (16.7286, 15.9398)
  line L16 (16.8757, 15.9398) -> (17.1667, 15.9398)
  spline S20 degree 2 poles (17.1667, 15.9398) (17.161, 16.0032) (17.1418, 16.1945) (17.1237, 16.2545) knots 0 0 0 1 2 2 2
  spline S21 degree 2 poles (17.1237, 16.2545) (17.1022, 16.3247) (17.0127, 16.4164) (16.9335, 16.4164) knots 0 0 0 1 2 2 2
  spline S22 degree 2 poles (16.9335, 16.4164) (16.8429, 16.4164) (16.7512, 16.3145) (16.7512, 16.2171) knots 0 0 0 1 2 2 2
  spline S23 degree 2 poles (16.7512, 16.2171) (16.7512, 16.1345) (16.8225, 15.9986) (16.8757, 15.9398) knots 0 0 0 1 2 2 2
  line L17 (17.4769, 14.9594) -> (17.4769, 14.9684)
  spline S24 degree 2 poles (17.4769, 14.9684) (17.4825, 14.9888) (17.4848, 15.0329) (17.4848, 15.0635) knots 0 0 0 1 2 2 2
  spline S25 degree 2 poles (17.4848, 15.0635) (17.4848, 15.1348) (17.4225, 15.2752) (17.3614, 15.3386) knots 0 0 0 1 2 2 2
  line L18 (17.3614, 15.3386) -> (16.6176, 15.3386)
  line L19 (16.6176, 15.3386) -> (16.6176, 15.5152)
  line L20 (16.6176, 15.5152) -> (17.6659, 15.5152)
  line L21 (17.6659, 15.5152) -> (17.6659, 15.3386)
  line L22 (17.6659, 15.3386) -> (17.5097, 15.3386)
  spline S26 degree 2 poles (17.5097, 15.3386) (17.5957, 15.2424) (17.6659, 15.0986) (17.6659, 15.0307) knots 0 0 0 1 2 2 2
  spline S27 degree 2 poles (17.6659, 15.0307) (17.6659, 15.0035) (17.6637, 14.9763) (17.6603, 14.9594) knots 0 0 0 1 2 2 2
  line L23 (17.6603, 14.9594) -> (17.4769, 14.9594)
  spline S28 degree 2 poles (16.5927, 14.5394) (16.5927, 14.6446) (16.6493, 14.8269) (16.681, 14.8869) knots 0 0 0 1 2 2 2
  line L24 (16.681, 14.8869) -> (16.8791, 14.8869)
  line L25 (16.8791, 14.8869) -> (16.8791, 14.8779)
  spline S29 degree 2 poles (16.8791, 14.8779) (16.861, 14.8552) (16.818, 14.7941) (16.7942, 14.7431) knots 0 0 0 1 2 2 2
  spline S30 degree 2 poles (16.7942, 14.7431) (16.7727, 14.699) (16.741, 14.5903) (16.741, 14.5326) knots 0 0 0 1 2 2 2
  spline S31 degree 2 poles (16.741, 14.5326) (16.741, 14.4907) (16.7603, 14.3945) (16.7761, 14.3718) knots 0 0 0 1 2 2 2
  spline S32 degree 2 poles (16.7761, 14.3718) (16.7976, 14.339) (16.8463, 14.3095) (16.8961, 14.3095) knots 0 0 0 1 2 2 2
  spline S33 degree 2 poles (16.8961, 14.3095) (16.9584, 14.3095) (17.0229, 14.3775) (17.0444, 14.4646) knots 0 0 0 1 2 2 2
  spline S34 degree 2 poles (17.0444, 14.4646) (17.0523, 14.4986) (17.075, 14.6073) (17.0874, 14.6537) knots 0 0 0 1 2 2 2
  spline S35 degree 2 poles (17.0874, 14.6537) (17.1225, 14.7737) (17.2674, 14.8824) (17.3705, 14.8824) knots 0 0 0 1 2 2 2
  spline S36 degree 2 poles (17.3705, 14.8824) (17.5131, 14.8824) (17.6908, 14.6684) (17.6908, 14.4918) knots 0 0 0 1 2 2 2
  spline S37 degree 2 poles (17.6908, 14.4918) (17.6908, 14.4046) (17.6478, 14.228) (17.615, 14.168) knots 0 0 0 1 2 2 2
  line L26 (17.615, 14.168) -> (17.4259, 14.168)
  line L27 (17.4259, 14.168) -> (17.4259, 14.1771)
  spline S38 degree 2 poles (17.4259, 14.1771) (17.4803, 14.245) (17.5425, 14.4103) (17.5425, 14.4952) knots 0 0 0 1 2 2 2
  spline S39 degree 2 poles (17.5425, 14.4952) (17.5425, 14.5824) (17.469, 14.7024) (17.3954, 14.7024) knots 0 0 0 1 2 2 2
  spline S40 degree 2 poles (17.3954, 14.7024) (17.3286, 14.7024) (17.264, 14.6311) (17.2437, 14.5518) knots 0 0 0 1 2 2 2
  spline S41 degree 2 poles (17.2437, 14.5518) (17.2335, 14.5133) (17.2131, 14.416) (17.2006, 14.3628) knots 0 0 0 1 2 2 2
  spline S42 degree 2 poles (17.2006, 14.3628) (17.1712, 14.2473) (17.0365, 14.1295) (16.9199, 14.1295) knots 0 0 0 1 2 2 2
  spline S43 degree 2 poles (16.9199, 14.1295) (16.852, 14.1295) (16.732, 14.1827) (16.6878, 14.2348) knots 0 0 0 1 2 2 2
  spline S44 degree 2 poles (16.6878, 14.2348) (16.6414, 14.2903) (16.5927, 14.4318) (16.5927, 14.5394) knots 0 0 0 1 2 2 2
  line L28 (16.6176, 13.1424) -> (16.6176, 13.319)
  line L29 (16.6176, 13.319) -> (17.2154, 13.319)
  spline S45 degree 2 poles (17.2154, 13.319) (17.2878, 13.319) (17.4123, 13.3325) (17.4497, 13.3529) knots 0 0 0 1 2 2 2
  spline S46 degree 2 poles (17.4497, 13.3529) (17.4893, 13.3744) (17.5278, 13.4514) (17.5278, 13.5171) knots 0 0 0 1 2 2 2
  spline S47 degree 2 poles (17.5278, 13.5171) (17.5278, 13.5827) (17.4576, 13.722) (17.401, 13.7888) knots 0 0 0 1 2 2 2
  line L30 (17.401, 13.7888) -> (16.6176, 13.7888)
  line L31 (16.6176, 13.7888) -> (16.6176, 13.9654)
  line L32 (16.6176, 13.9654) -> (18.0769, 13.9654)
  line L33 (18.0769, 13.9654) -> (18.0769, 13.7888)
  line L34 (18.0769, 13.7888) -> (17.5493, 13.7888)
  spline S48 degree 2 poles (17.5493, 13.7888) (17.6207, 13.7095) (17.6954, 13.5567) (17.6954, 13.4707) knots 0 0 0 1 2 2 2
  spline S49 degree 2 poles (17.6954, 13.4707) (17.6954, 13.3167) (17.4916, 13.1424) (17.298, 13.1424) knots 0 0 0 1 2 2 2
  line L35 (17.298, 13.1424) -> (16.6176, 13.1424)
  line L36 (16.6176, 12.7144) -> (16.6176, 12.891)
  line L37 (16.6176, 12.891) -> (17.6659, 12.891)
  line L38 (17.6659, 12.891) -> (17.6659, 12.7144)
  line L39 (17.6659, 12.7144) -> (16.6176, 12.7144)
  line L40 (17.8403, 12.702) -> (17.8403, 12.9024)
  line L41 (17.8403, 12.9024) -> (18.0237, 12.9024)
  line L42 (18.0237, 12.9024) -> (18.0237, 12.702)
  line L43 (18.0237, 12.702) -> (17.8403, 12.702)
  line L44 (16.6176, 12.2752) -> (16.6176, 12.4518)
  line L45 (16.6176, 12.4518) -> (18.0769, 12.4518)
  line L46 (18.0769, 12.4518) -> (18.0769, 12.2752)
  line L47 (18.0769, 12.2752) -> (16.6176, 12.2752)
  spline S50 degree 2 poles (16.5927, 10.8567) (16.5927, 10.9925) (16.6844, 11.2223) (16.7761, 11.3061) knots 0 0 0 1 2 2 2
  spline S51 degree 2 poles (16.7761, 11.3061) (16.8667, 11.3899) (17.1384, 11.4816) (17.315, 11.4816) knots 0 0 0 1 2 2 2
  spline S52 degree 2 poles (17.315, 11.4816) (17.4905, 11.4816) (17.7508, 11.3921) (17.8471, 11.3072) knots 0 0 0 1 2 2 2
  spline S53 degree 2 poles (17.8471, 11.3072) (17.941, 11.2235) (18.0395, 10.9948) (18.0395, 10.8533) knots 0 0 0 1 2 2 2
  spline S54 degree 2 poles (18.0395, 10.8533) (18.0395, 10.7831) (18.0191, 10.6597) (18.0033, 10.6076) knots 0 0 0 1 2 2 2
  spline S55 degree 2 poles (18.0033, 10.6076) (17.9886, 10.5623) (17.9467, 10.4684) (17.9218, 10.4219) knots 0 0 0 1 2 2 2
  line L48 (17.9218, 10.4219) -> (17.6976, 10.4219)
  line L49 (17.6976, 10.4219) -> (17.6976, 10.4367)
  spline S56 degree 2 poles (17.6976, 10.4367) (17.7203, 10.4616) (17.7837, 10.5385) (17.8142, 10.594) knots 0 0 0 1 2 2 2
  spline S57 degree 2 poles (17.8142, 10.594) (17.8437, 10.6472) (17.881, 10.7729) (17.881, 10.8544) knots 0 0 0 1 2 2 2
  spline S58 degree 2 poles (17.881, 10.8544) (17.881, 10.9438) (17.8074, 11.1035) (17.7373, 11.1635) knots 0 0 0 1 2 2 2
  spline S59 degree 2 poles (17.7373, 11.1635) (17.6659, 11.2223) (17.4497, 11.288) (17.315, 11.288) knots 0 0 0 1 2 2 2
  spline S60 degree 2 poles (17.315, 11.288) (17.1712, 11.288) (16.964, 11.2189) (16.8927, 11.1589) knots 0 0 0 1 2 2 2
  spline S61 degree 2 poles (16.8927, 11.1589) (16.8237, 11.1001) (16.7535, 10.9427) (16.7535, 10.8544) knots 0 0 0 1 2 2 2
  spline S62 degree 2 poles (16.7535, 10.8544) (16.7535, 10.774) (16.7931, 10.637) (16.8225, 10.5838) knots 0 0 0 1 2 2 2
  spline S63 degree 2 poles (16.8225, 10.5838) (16.852, 10.5329) (16.9131, 10.457) (16.9346, 10.4355) knots 0 0 0 1 2 2 2
  line L50 (16.9346, 10.4355) -> (16.9346, 10.4219)
  line L51 (16.9346, 10.4219) -> (16.7127, 10.4219)
  spline S64 degree 2 poles (16.7127, 10.4219) (16.6912, 10.4684) (16.6516, 10.5499) (16.6335, 10.6076) knots 0 0 0 1 2 2 2
  spline S65 degree 2 poles (16.6335, 10.6076) (16.6131, 10.6687) (16.5927, 10.7729) (16.5927, 10.8567) knots 0 0 0 1 2 2 2
  spline S66 degree 2 poles (17.1418, 9.4008) (16.8769, 9.4008) (16.5882, 9.6555) (16.5882, 9.8684) knots 0 0 0 1 2 2 2
  spline S67 degree 2 poles (16.5882, 9.8684) (16.5882, 10.0868) (16.8859, 10.337) (17.1418, 10.337) knots 0 0 0 1 2 2 2
  spline S68 degree 2 poles (17.1418, 10.337) (17.4044, 10.337) (17.6954, 10.0789) (17.6954, 9.8684) knots 0 0 0 1 2 2 2
  spline S69 degree 2 poles (17.6954, 9.8684) (17.6954, 9.6555) (17.4056, 9.4008) (17.1418, 9.4008) knots 0 0 0 1 2 2 2
  spline S70 degree 2 poles (17.1418, 9.5831) (17.3456, 9.5831) (17.5437, 9.7314) (17.5437, 9.8684) knots 0 0 0 1 2 2 2
  spline S71 degree 2 poles (17.5437, 9.8684) (17.5437, 10.0053) (17.3456, 10.1548) (17.1418, 10.1548) knots 0 0 0 1 2 2 2
  spline S72 degree 2 poles (17.1418, 10.1548) (16.9437, 10.1548) (16.7399, 10.0053) (16.7399, 9.8684) knots 0 0 0 1 2 2 2
  spline S73 degree 2 poles (16.7399, 9.8684) (16.7399, 9.7325) (16.9403, 9.5831) (17.1418, 9.5831) knots 0 0 0 1 2 2 2
  line L52 (16.6176, 8.9457) -> (16.6176, 9.1699)
  line L53 (16.6176, 9.1699) -> (16.8848, 9.1699)
  line L54 (16.8848, 9.1699) -> (16.8848, 8.9457)
  line L55 (16.8848, 8.9457) -> (16.6176, 8.9457)
  spline S74 degree 2 poles (15.2934, 19.7606) (15.2028, 19.7606) (15.0398, 19.8251) (14.9832, 19.8828) knots 0 0 0 1 2 2 2
  spline S75 degree 2 poles (14.9832, 19.8828) (14.9118, 19.9553) (14.8383, 20.1511) (14.8383, 20.3006) knots 0 0 0 1 2 2 2
  line L56 (14.8383, 20.3006) -> (14.8383, 20.4579)
  line L57 (14.8383, 20.4579) -> (14.3175, 20.4579)
  line L58 (14.3175, 20.4579) -> (14.3175, 20.6436)
  line L59 (14.3175, 20.6436) -> (15.7145, 20.6436)
  line L60 (15.7145, 20.6436) -> (15.7145, 20.2926)
  spline S76 degree 2 poles (15.7145, 20.2926) (15.7145, 20.1681) (15.6737, 19.9938) (15.6273, 19.927) knots 0 0 0 1 2 2 2
  spline S77 degree 2 poles (15.6273, 19.927) (15.5741, 19.8489) (15.41, 19.7606) (15.2934, 19.7606) knots 0 0 0 1 2 2 2
  spline S78 degree 2 poles (15.2877, 19.9541) (15.3602, 19.9541) (15.4666, 20.004) (15.5005, 20.0549) knots 0 0 0 1 2 2 2
  spline S79 degree 2 poles (15.5005, 20.0549) (15.53, 20.0991) (15.5537, 20.2168) (15.5537, 20.304) knots 0 0 0 1 2 2 2
  line L61 (15.5537, 20.304) -> (15.5537, 20.4579)
  line L62 (15.5537, 20.4579) -> (14.9967, 20.4579)
  line L63 (14.9967, 20.4579) -> (14.9967, 20.3311)
  spline S80 degree 2 poles (14.9967, 20.3311) (14.9967, 20.2179) (15.033, 20.0787) (15.0805, 20.0334) knots 0 0 0 1 2 2 2
  spline S81 degree 2 poles (15.0805, 20.0334) (15.1224, 19.9915) (15.2209, 19.9541) (15.2877, 19.9541) knots 0 0 0 1 2 2 2
  spline S82 degree 2 poles (14.4284, 19.0134) (14.4126, 19.0349) (14.356, 19.1073) (14.339, 19.1413) knots 0 0 0 1 2 2 2
  spline S83 degree 2 poles (14.339, 19.1413) (14.3141, 19.1877) (14.2881, 19.2749) (14.2881, 19.3541) knots 0 0 0 1 2 2 2
  spline S84 degree 2 poles (14.2881, 19.3541) (14.2881, 19.4187) (14.3367, 19.5353) (14.3809, 19.5794) knots 0 0 0 1 2 2 2
  spline S85 degree 2 poles (14.3809, 19.5794) (14.4239, 19.6213) (14.5507, 19.6723) (14.6209, 19.6723) knots 0 0 0 1 2 2 2
  spline S86 degree 2 poles (14.6209, 19.6723) (14.7296, 19.6723) (14.8835, 19.5806) (14.9277, 19.4809) knots 0 0 0 1 2 2 2
  spline S87 degree 2 poles (14.9277, 19.4809) (14.9684, 19.3926) (14.999, 19.1526) (15.0069, 19.0134) knots 0 0 0 1 2 2 2
  line L64 (15.0069, 19.0134) -> (15.0409, 19.0134)
  spline S88 degree 2 poles (15.0409, 19.0134) (15.102, 19.0134) (15.1779, 19.0507) (15.1994, 19.0847) knots 0 0 0 1 2 2 2
  spline S89 degree 2 poles (15.1994, 19.0847) (15.2209, 19.1187) (15.2345, 19.216) (15.2345, 19.2681) knots 0 0 0 1 2 2 2
  spline S90 degree 2 poles (15.2345, 19.2681) (15.2345, 19.3292) (15.1983, 19.4945) (15.1632, 19.5772) knots 0 0 0 1 2 2 2
  line L65 (15.1632, 19.5772) -> (15.1632, 19.5874)
  line L66 (15.1632, 19.5874) -> (15.3432, 19.5874)
  spline S91 degree 2 poles (15.3432, 19.5874) (15.3568, 19.5387) (15.3907, 19.3564) (15.3907, 19.267) knots 0 0 0 1 2 2 2
  spline S92 degree 2 poles (15.3907, 19.267) (15.3907, 19.1583) (15.3568, 19.01) (15.3126, 18.9511) knots 0 0 0 1 2 2 2
  spline S93 degree 2 poles (15.3126, 18.9511) (15.2696, 18.8934) (15.1326, 18.8368) (15.0341, 18.8368) knots 0 0 0 1 2 2 2
  line L67 (15.0341, 18.8368) -> (14.3175, 18.8368)
  line L68 (14.3175, 18.8368) -> (14.3175, 19.0134)
  line L69 (14.3175, 19.0134) -> (14.4284, 19.0134)
  line L70 (14.5756, 19.0134) -> (14.8666, 19.0134)
  spline S94 degree 2 poles (14.8666, 19.0134) (14.8609, 19.0768) (14.8417, 19.2681) (14.8235, 19.3281) knots 0 0 0 1 2 2 2
  spline S95 degree 2 poles (14.8235, 19.3281) (14.802, 19.3983) (14.7126, 19.49) (14.6333, 19.49) knots 0 0 0 1 2 2 2
  spline S96 degree 2 poles (14.6333, 19.49) (14.5428, 19.49) (14.4511, 19.3881) (14.4511, 19.2907) knots 0 0 0 1 2 2 2
  spline S97 degree 2 poles (14.4511, 19.2907) (14.4511, 19.2081) (14.5224, 19.0722) (14.5756, 19.0134) knots 0 0 0 1 2 2 2
  line L71 (15.1768, 18.033) -> (15.1768, 18.042)
  spline S98 degree 2 poles (15.1768, 18.042) (15.1824, 18.0624) (15.1847, 18.1066) (15.1847, 18.1371) knots 0 0 0 1 2 2 2
  spline S99 degree 2 poles (15.1847, 18.1371) (15.1847, 18.2085) (15.1224, 18.3488) (15.0613, 18.4122) knots 0 0 0 1 2 2 2
  line L72 (15.0613, 18.4122) -> (14.3175, 18.4122)
  line L73 (14.3175, 18.4122) -> (14.3175, 18.5888)
  line L74 (14.3175, 18.5888) -> (15.3658, 18.5888)
  line L75 (15.3658, 18.5888) -> (15.3658, 18.4122)
  line L76 (15.3658, 18.4122) -> (15.2096, 18.4122)
  spline S100 degree 2 poles (15.2096, 18.4122) (15.2956, 18.316) (15.3658, 18.1722) (15.3658, 18.1043) knots 0 0 0 1 2 2 2
  spline S101 degree 2 poles (15.3658, 18.1043) (15.3658, 18.0771) (15.3635, 18.05) (15.3602, 18.033) knots 0 0 0 1 2 2 2
  line L77 (15.3602, 18.033) -> (15.1768, 18.033)
  spline S102 degree 2 poles (14.2971, 17.579) (14.2971, 17.7228) (14.4613, 17.8847) (14.639, 17.8847) knots 0 0 0 1 2 2 2
  line L78 (14.639, 17.8847) -> (15.2198, 17.8847)
  line L79 (15.2198, 17.8847) -> (15.2198, 18.0036)
  line L80 (15.2198, 18.0036) -> (15.3658, 18.0036)
  line L81 (15.3658, 18.0036) -> (15.3658, 17.8847)
  line L82 (15.3658, 17.8847) -> (15.6669, 17.8847)
  line L83 (15.6669, 17.8847) -> (15.6669, 17.7081)
  line L84 (15.6669, 17.7081) -> (15.3658, 17.7081)
  line L85 (15.3658, 17.7081) -> (15.3658, 17.3832)
  line L86 (15.3658, 17.3832) -> (15.2198, 17.3832)
  line L87 (15.2198, 17.3832) -> (15.2198, 17.7081)
  line L88 (15.2198, 17.7081) -> (14.7205, 17.7081)
  spline S103 degree 2 poles (14.7205, 17.7081) (14.6413, 17.7081) (14.5541, 17.7024) (14.5167, 17.6832) knots 0 0 0 1 2 2 2
  spline S104 degree 2 poles (14.5167, 17.6832) (14.4839, 17.6673) (14.4511, 17.596) (14.4511, 17.5349) knots 0 0 0 1 2 2 2
  spline S105 degree 2 poles (14.4511, 17.5349) (14.4511, 17.4919) (14.4771, 17.4115) (14.485, 17.3934) knots 0 0 0 1 2 2 2
  line L89 (14.485, 17.3934) -> (14.485, 17.3832)
  line L90 (14.485, 17.3832) -> (14.3266, 17.3832)
  spline S106 degree 2 poles (14.3266, 17.3832) (14.313, 17.433) (14.2971, 17.5349) (14.2971, 17.579) knots 0 0 0 1 2 2 2
  line L91 (14.3175, 15.6398) -> (14.3175, 15.8481)
  line L92 (14.3175, 15.8481) -> (15.522, 16.4662)
  line L93 (15.522, 16.4662) -> (14.3175, 16.4662)
  line L94 (14.3175, 16.4662) -> (14.3175, 16.6394)
  line L95 (14.3175, 16.6394) -> (15.7145, 16.6394)
  line L96 (15.7145, 16.6394) -> (15.7145, 16.3756)
  line L97 (15.7145, 16.3756) -> (14.6084, 15.813)
  line L98 (14.6084, 15.813) -> (15.7145, 15.813)
  line L99 (15.7145, 15.813) -> (15.7145, 15.6398)
  line L100 (15.7145, 15.6398) -> (14.3175, 15.6398)
  spline S107 degree 2 poles (14.8417, 14.5088) (14.5767, 14.5088) (14.2881, 14.7635) (14.2881, 14.9763) knots 0 0 0 1 2 2 2
  spline S108 degree 2 poles (14.2881, 14.9763) (14.2881, 15.1948) (14.5858, 15.445) (14.8417, 15.445) knots 0 0 0 1 2 2 2
  spline S109 degree 2 poles (14.8417, 15.445) (15.1043, 15.445) (15.3952, 15.1869) (15.3952, 14.9763) knots 0 0 0 1 2 2 2
  spline S110 degree 2 poles (15.3952, 14.9763) (15.3952, 14.7635) (15.1054, 14.5088) (14.8417, 14.5088) knots 0 0 0 1 2 2 2
  spline S111 degree 2 poles (14.8417, 14.6911) (15.0454, 14.6911) (15.2435, 14.8394) (15.2435, 14.9763) knots 0 0 0 1 2 2 2
  spline S112 degree 2 poles (15.2435, 14.9763) (15.2435, 15.1133) (15.0454, 15.2628) (14.8417, 15.2628) knots 0 0 0 1 2 2 2
  spline S113 degree 2 poles (14.8417, 15.2628) (14.6435, 15.2628) (14.4398, 15.1133) (14.4398, 14.9763) knots 0 0 0 1 2 2 2
  spline S114 degree 2 poles (14.4398, 14.9763) (14.4398, 14.8405) (14.6401, 14.6911) (14.8417, 14.6911) knots 0 0 0 1 2 2 2
  line L101 (14.3175, 14.0537) -> (14.3175, 14.2778)
  line L102 (14.3175, 14.2778) -> (14.5847, 14.2778)
  line L103 (14.5847, 14.2778) -> (14.5847, 14.0537)
  line L104 (14.5847, 14.0537) -> (14.3175, 14.0537)
  line L105 (14.3175, 12.3103) -> (14.3175, 13.1718)
  line L106 (14.3175, 13.1718) -> (14.5156, 13.1718)
  spline S115 degree 2 poles (14.5156, 13.1718) (14.6028, 13.079) (14.7647, 12.9137) (14.8518, 12.8344) knots 0 0 0 1 2 2 2
  spline S116 degree 2 poles (14.8518, 12.8344) (15.0273, 12.6748) (15.2379, 12.5582) (15.35, 12.5582) knots 0 0 0 1 2 2 2
  spline S117 degree 2 poles (15.35, 12.5582) (15.4088, 12.5582) (15.4971, 12.5944) (15.5254, 12.6273) knots 0 0 0 1 2 2 2
  spline S118 degree 2 poles (15.5254, 12.6273) (15.5537, 12.6601) (15.582, 12.7461) (15.582, 12.7982) knots 0 0 0 1 2 2 2
  spline S119 degree 2 poles (15.582, 12.7982) (15.582, 12.848) (15.5571, 12.9499) (15.5379, 12.9963) knots 0 0 0 1 2 2 2
  spline S120 degree 2 poles (15.5379, 12.9963) (15.522, 13.0359) (15.4768, 13.1095) (15.4609, 13.1322) knots 0 0 0 1 2 2 2
  line L107 (15.4609, 13.1322) -> (15.4609, 13.1424)
  line L108 (15.4609, 13.1424) -> (15.6602, 13.1424)